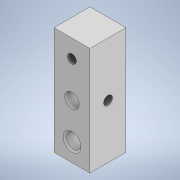
# Autodesk Inventor part: 3SR05_振子固定パーツA
Saved by Autodesk Inventor 2021 (Build 250183000, 183)
## iProperties
Created: 2021-04-20
Part Number: 3SR05_振子固定パーツA
Material: 一般
Document SubType Name: Modeling
Designer: ryusei
Density: 1 g/cm^3
Appearance: 既定
Author: ryusei
Autodesk Inventor part; units mm, degrees
ref_plane "YZ Plane" through (0, 0, 0) normal (1, 0, 0) x (0, 1, 0)
ref_plane "XZ Plane" through (0, 0, 0) normal (0, 1, 0) x (-1, 0, 0)
ref_plane "XY Plane" through (0, 0, 0) normal (0, 0, 1) x (1, 0, 0)
sketch "スケッチ1" plane through (0, 0, 0) normal (0, 0, 1) x (1, 0, 0)
  line L0 (0, 0) -> (10, 0)
  line L1 (10, 0) -> (10, 30)
  line L2 (10, 30) -> (0, 30)
  line L3 (0, 30) -> (0, 0)
  dimension "d0" = 10
  dimension "d1" = 30
  constraints: 8 end point, 2 parallel, 1 horizontal, 1 perpendicular
  measures "d0" distance between parallel lines of L1 L3
  measures "d1" distance between parallel lines of L0 L2
extrude "押し出し1" add sketch "スケッチ1" along normal blind 10
sketch "スケッチ2" plane through (0, 0, 10) normal (0, 0, 1) x (1, 0, 0)
  line L0 (10, 30) -> (0, 30) projected
  line L1 (10, 0) -> (10, 30) projected
  point P0 (0, 0)
  point P1 (5, 15)
  dimension "d4" = 15
  dimension "d5" = 5
  measures "d4" distance from line of L0 point (5, 15)
  measures "d5" distance from line of L1 point (5, 15)
hole "穴1" at (5, 15, 10) direction (0, 0, -1) diameter 4 end through all
sketch "スケッチ3" plane through (0, 0, 10) normal (0, 0, 1) x (1, 0, 0)
  point P0 (0, 0)
sketch "スケッチ4" plane through (0, 0, 10) normal (0, 0, 1) x (1, 0, 0)
  line L0 (10, 30) -> (0, 30) projected
  line L1 (10, 0) -> (10, 30) projected
  point P0 (0, 0)
  point P1 (5, 25)
  dimension "d13" = 5
  dimension "d14" = 5
  measures "d13" distance from line of L0 point (5, 25)
  measures "d14" distance from line of L1 point (5, 25)
hole "穴2" at (5, 25, 10) direction (0, 0, -1) diameter 2.459 end through all thread size "M3x0.5" class "6H" standard "ANSI Metric M Profile"
sketch "スケッチ6" plane through (10, 0, 0) normal (1, 0, 0) x (0, 0, -1)
  line L0 (0, 0) -> (0, 30) projected
  line L1 (0, 30) -> (-10, 30) projected
  point P0 (-5, 15)
  dimension "d31" = 5
  dimension "d32" = 15
  measures "d31" distance from line of L0 point (-5, 15)
  measures "d32" distance from line of point (-5, 15) L1
hole "穴4" at (10, 15, 5) direction (-1, 0, 0) diameter 2.459 end through all thread size "M3x0.5" class "6H" standard "ANSI Metric M Profile"
sketch "スケッチ8" plane through (0, 0, 10) normal (0, 0, 1) x (1, 0, 0)
  line L0 (10, 0) -> (10, 30) projected
  line L1 (0, 0) -> (10, 0) projected
  point P0 (5, 5)
  dimension "d49" = 5
  dimension "d50" = 5
  measures "d49" distance from line of L0 point (5, 5)
  measures "d50" distance from line of L1 point (5, 5)
hole "穴6" at (5, 5, 10) direction (0, 0, -1) diameter 4 depth 10 tip angle 118 countersink diameter 5 countersink angle 90
